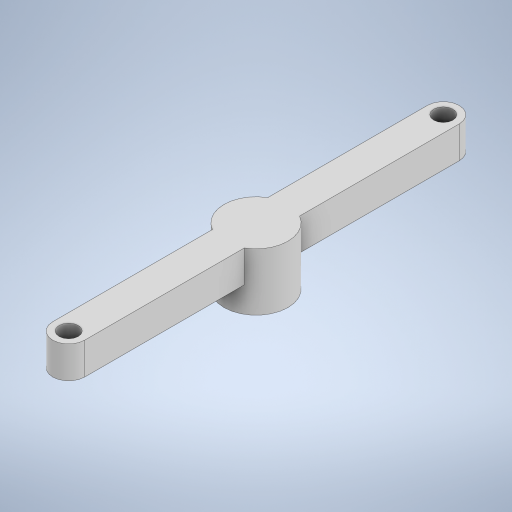
# Autodesk Inventor part: gripper_mechanism
Saved by Autodesk Inventor 2023 (Build 270158000, 158)
## iProperties
Created: 2024-06-26
Part Number: gripper_mechanism
Material: Generic
Document SubType Name: Modeling
Designer: Swoby
Density: 1 g/cm^3
Appearance: Default
Author: Swoby
Autodesk Inventor part; units mm, degrees
ref_plane "YZ Plane" through (0, 0, 0) normal (1, 0, 0) x (0, 1, 0)
ref_plane "XZ Plane" through (0, 0, 0) normal (0, 1, 0) x (-1, 0, 0)
ref_plane "XY Plane" through (0, 0, 0) normal (0, 0, 1) x (1, 0, 0)
sketch "Sketch1" plane through (0, 0, 0) normal (0, 1, 0) x (-1, 0, 0)
  circle A0 centre (0, 0) radius 5
  line L0 (2.5, 4.3301) -> (2.5, -4.3301)
  line L1 (-2.5, 4.3301) -> (-2.5, -4.3301)
  line L2 (-2.5, 4.3301) -> (-2.5, -4.3301)
  line L3 (-2.5, 4.3301) -> (-2.5, 29.3301)
  line L4 (-2.5, -4.3301) -> (-2.5, -29.3301)
  line L5 (2.5, -4.3301) -> (2.5, -29.3301)
  arc A1 (-2.5, -29.3301) -> (2.5, -29.3301) centre (0, -29.3301) ccw
  line L6 (2.5, 4.3301) -> (2.5, 29.3301)
  arc A2 (2.5, 29.3301) -> (-2.5, 29.3301) centre (0, 29.3301) ccw
  circle A3 centre (0, 29.3301) radius 1.5
  circle A4 centre (0, -29.3301) radius 1.5
  dimension "d0" = 10
  dimension "d1" = 5
  dimension "d2" = 2.5
  dimension "d18" = 25
  dimension "d19" = 25
  dimension "d20" = 25
  dimension "d21" = 3
  dimension "d22" = 3
  dimension "d23" = 25
  dimension "d24" = 2.5
  constraints: 14 end point, 8 point on circle, 5 centre point, 3 coincident, 3 tangent, 2 point on line, 2 vertical, 1 parallel
  measures "d0" diameter of A0
  measures "d1" distance between parallel lines of L1 L0
  measures "d2" distance from line of L0 point (0, 0)
  measures "d18" distance of L1.end L4.end
  measures "d19" distance of L2.start L3.end
  measures "d20" distance of L0.start L6.end
  measures "d21" diameter of A3
  measures "d22" diameter of A4
  measures "d23" distance of L0.end L5.end
  measures "d24" radius of A2
extrude "Extrusion1" add sketch "Sketch1" along normal blind 5
sketch "Sketch2" plane through (0, 0, 0) normal (0, -1, 0) x (1, 0, 0)
  circle A0 centre (0, 0) radius 5
  circle A1 centre (0, 0) radius 2.5
  dimension "d14" = 5
  dimension "d15" = 10
  constraints: 2 centre point, 2 coincident
  measures "d14" diameter of A1
  measures "d15" diameter of A0
extrude "Extrusion2" add sketch "Sketch2" along normal blind 4
equation "\"d2\" = 0.5 * d1"
body "Solid1"
